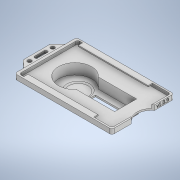
# Autodesk Inventor part: badge
Saved by Autodesk Inventor 2020 (Build 240168000, 168)
## iProperties
Created: 2019-12-22
Part Number: badge
Material: Generic
Document SubType Name: Modeling
Designer: user
Density: 1 g/cm^3
Appearance: Default
Author: user
## iProperties of the stored document _3DPrint.ipt
Created: 2019-12-23
Part Number: _3DPrint
Material: Generic
Document SubType Name: Modeling
Designer: user
Density: 1 g/cm^3
Appearance: Default
Author: user
Autodesk Inventor part; units mm, degrees
ref_plane "YZ Plane" through (0, 0, 0) normal (1, 0, 0) x (0, 1, 0)
ref_plane "XZ Plane" through (0, 0, 0) normal (0, 1, 0) x (-1, 0, 0)
ref_plane "XY Plane" through (0, 0, 0) normal (0, 0, 1) x (1, 0, 0)
sketch "Sketch1" plane through (0, 0, 0) normal (0, 1, 0) x (-1, 0, 0)
  line L0 (11.118, 24.1263) -> (-75.7851, 24.1263)
  line L1 (-75.7851, -33.7737) -> (11.118, -33.7737)
  line L2 (13.118, 15.5763) -> (20.4648, 8.8849)
  line L3 (21.118, 7.4063) -> (21.118, -16.3891)
  line L4 (20.5328, -17.8027) -> (13.118, -25.2237)
  line L5 (18.618, -9.3889) -> (18.618, 0.3517)
  circle A0 centre (-14.3851, -4.8237) radius 17
  line L6 (-63.1708, 4.9263) -> (-63.1708, -14.5737)
  line L7 (-61.1708, -16.5737) -> (-26.6708, -16.5737)
  line L8 (-26.6708, 6.9263) -> (-61.1708, 6.9263)
  arc A1 (-63.1708, -14.5737) -> (-61.1708, -16.5737) centre (-61.1708, -14.5737) ccw
  arc A2 (-61.1708, 6.9263) -> (-63.1708, 4.9263) centre (-61.1708, 4.9263) ccw
  line L9 (-29.1351, -0.5737) -> (-55.6708, -0.5737)
  line L10 (-55.6708, -0.5737) -> (-55.6708, -9.0737)
  line L11 (-55.6708, -9.0737) -> (-29.1351, -9.0737)
  line L12 (-29.1351, -9.0737) -> (-29.1351, -0.5737)
  line L13 (-77.7851, 6.1263) -> (-77.7851, 22.1263)
  line L14 (-77.7851, -15.7737) -> (-77.7851, -31.7737)
  line L15 (8.6149, 22.6263) -> (-74.2851, 22.6263)
  line L16 (-74.2851, -32.2737) -> (8.6149, -32.2737)
  line L17 (10.6149, -30.2737) -> (10.6149, 20.6263)
  line L18 (-76.2851, 20.6263) -> (-76.2851, 4.8009)
  line L19 (-76.2851, -30.2737) -> (-76.2851, -14.4482)
  line L20 (13.118, 22.1263) -> (13.118, 15.5763)
  line L21 (13.118, -25.2237) -> (13.118, -31.7737)
  arc A3 (-77.7851, -31.7737) -> (-75.7851, -33.7737) centre (-75.7851, -31.7737) ccw
  arc A4 (-76.2851, -30.2737) -> (-74.2851, -32.2737) centre (-74.2851, -30.2737) ccw
  arc A5 (-74.2851, 22.6263) -> (-76.2851, 20.6263) centre (-74.2851, 20.6263) ccw
  arc A6 (-75.7851, 24.1263) -> (-77.7851, 22.1263) centre (-75.7851, 22.1263) ccw
  arc A7 (13.118, 22.1263) -> (11.118, 24.1263) centre (11.118, 22.1263) ccw
  arc A8 (10.6149, 20.6263) -> (8.6149, 22.6263) centre (8.6149, 20.6263) ccw
  arc A9 (8.6149, -32.2737) -> (10.6149, -30.2737) centre (8.6149, -30.2737) ccw
  arc A10 (11.118, -33.7737) -> (13.118, -31.7737) centre (11.118, -31.7737) ccw
  arc A11 (20.5328, -17.8027) -> (21.118, -16.3891) centre (19.118, -16.3891) ccw
  arc A12 (21.118, 7.4063) -> (20.4648, 8.8849) centre (19.118, 7.4063) ccw
  arc A13 (-77.7851, -15.7737) -> (-77.7851, 6.1263) centre (-86.1254, -4.8237) ccw
  circle A14 centre (17.118, 6.2771) radius 1.8024
  circle A15 centre (17.118, -15.3502) radius 1.8024
  line L22 (13.118, 15.5763) -> (13.118, -25.2237)
  arc A16 (18.618, 0.3517) -> (15.618, 0.3153) centre (17.1248, -0.2229) ccw
  line L23 (15.618, 0.3153) -> (15.618, -9.4244)
  arc A17 (15.618, -9.4244) -> (18.618, -9.3889) centre (17.1115, -8.8502) ccw
  point P0 (0, 0)
  point P1 (13.118, 24.1263)
  point P2 (-77.7851, -33.7737)
  point P3 (-77.7851, 24.1263)
  point P4 (13.118, -33.7737)
  point P5 (21.118, -17.217)
  point P6 (-63.1708, -16.5737)
  dimension "d19" = 18
  dimension "d20" = 34
  dimension "d26" = 2
  dimension "d28" = 7.5
  dimension "d32" = 7.5
  dimension "d33" = 7.5
  dimension "d36" = 1.5
  dimension "d37" = 1.5
  dimension "d40" = 1.5
  dimension "d41" = 2
  dimension "d84" = 54.9
  dimension "d89" = 18
  dimension "d106" = 8
  dimension "d110" = 13.7646
  dimension "d116" = 1.5
  dimension "d122" = 3.6047
  dimension "d123" = 3.6047
  dimension "d155" = 25
  dimension "d163" = 15.7
  dimension "d164" = 15.7
  dimension "d165" = 27.45
  dimension "d166" = 27.45
  dimension "d167" = 8.5
  dimension "d171" = 26.5357
  dimension "d173" = 39.75
  dimension "d174" = 2.5032
  dimension "d177" = 86.9
  dimension "d182" = 4
  dimension "d183" = 4
  dimension "d187" = 3
  dimension "d188" = 1.6
  dimension "d189" = 1.6
  dimension "d190" = 2.5
  dimension "d191" = 2.5
  dimension "d192" = 8
  dimension "d193" = 6.5
  dimension "d194" = 6.5
  dimension "d195" = 6.55
  dimension "d196" = 6.55
  dimension "d202" = 15.7993
  dimension "d203" = 15.7993
  dimension "d204" = 23.7954
  dimension "d208" = 11.8273
  constraints: 48 end point, 34 point on circle, 24 tangent, 18 centre point, 13 point on line, 10 equal radius, 7 equal length, 5 vertical, 3 horizontal, 3 perpendicular
  measures "d19" distance of point (-77.785, 24.126) L13.start
  measures "d20" diameter of A0
  measures "d26" radius of A1
  measures "d28" distance between parallel lines of L7 L11
  measures "d32" distance between parallel lines of L9 L8
  measures "d33" distance between parallel lines of L6 L10
  measures "d36" distance between parallel lines of L0 L15
  measures "d37" distance between parallel lines of L1 L16
  measures "d40" distance between parallel lines of L14 L19
  measures "d41" radius of A3
  measures "d84" distance between parallel lines of L16 L15
  measures "d89" distance of L14.start point (-77.785, -33.774)
  measures "d106" distance between parallel lines of L20 L3
  measures "d110" radius of A13
  measures "d116" distance between parallel lines of L18 L13
  measures "d122" diameter of A15
  measures "d123" diameter of A14
  measures "d155" distance from line of L17 A0.centre
  measures "d163" distance between parallel lines of L16 L7
  measures "d164" distance between parallel lines of L15 L8
  measures "d165" distance from line of L16 A0.centre
  measures "d166" distance from line of L15 A0.centre
  measures "d167" distance between parallel lines of L9 L11
  measures "d171" distance between parallel lines of L10 L12
  measures "d173" distance between parallel lines of L17 L12
  measures "d174" distance between parallel lines of L17 L21
  measures "d177" distance between parallel lines of L19 L17
  measures "d182" distance from line of L22 A14.centre
  measures "d183" distance from line of L22 A15.centre
  measures "d187" distance between parallel lines of L23 L5
  measures "d188" radius of A16
  measures "d189" radius of A17
  measures "d190" distance between parallel lines of L3 L5
  measures "d191" distance between parallel lines of L22 L23
  measures "d192" distance between parallel lines of L22 L3
  measures "d193" distance of A14.centre A16.centre
  measures "d194" distance of A15.centre A17.centre
  measures "d195" distance of L20.start L2.start
  measures "d196" distance of L21.end L4.end
  measures "d202" vertical distance of L4.end L23.end
  measures "d203" vertical distance of L2.start A16.centre
  measures "d204" distance of L3.end L3.start
extrude "OutsideFrame_Ex" add sketch "Sketch1" along normal blind 4.5 contours A7 L20 L22 L21 A10 L1 A3 L14 A13 L19 A4 L16 A9 L17 A8 L15 A5 L18 L13 A6 L0
extrude "CardRidge" add sketch "Sketch1" along normal blind 1.5 contours L18 A5 L15 A8 L17 A9 L16 A4 L19 A13
extrude "TokenBuffer" add sketch "Sketch1" against normal blind 10 contours A0 L11 L12 L9 | A0 L9 L10 L11 L7 A1 L6 A2 L8 picked at (-18.5518, -4.8237)
sketch "Sketch4" plane through (0, 0, 0) normal (0, 1, 0) x (1, 0, 0)
  arc A0 (26.6708, 16.5737) -> (26.6708, -6.9263) centre (14.3851, 4.8237) ccw projected
  circle A1 centre (14.3851, 4.8237) radius 15.5
  line L0 (26.0122, -5.4263) -> (61.6708, -5.4263)
  line L1 (61.6708, -5.4263) -> (61.6708, 15.0737)
  line L2 (61.6708, 15.0737) -> (26.0122, 15.0737)
  line L3 (26.0122, 15.0737) -> (26.0122, -5.4263)
  line L4 (61.1708, -6.9263) -> (26.6708, -6.9263) projected
  line L5 (26.6708, 16.5737) -> (61.1708, 16.5737) projected
  line L6 (63.1708, 14.5737) -> (63.1708, -4.9263) projected
  point P0 (0, 0)
  point P1 (26.0122, 15.0737)
  point P2 (26.0122, 15.0737)
  dimension "d56" = 1.5
  dimension "d57" = 1.5
  dimension "d58" = 1.5
  dimension "d59" = 1.5
  constraints: 8 end point, 2 parallel, 1 coincident, 1 horizontal, 1 perpendicular, 3 other
  measures "d57" distance between parallel lines of L4 L0
  measures "d58" distance between parallel lines of L5 L2
  measures "d59" distance between parallel lines of L6 L1
extrude "TokenCut" cut sketch "Sketch4" against normal blind 8.5
sketch "Sketch5" plane through (74.2851, 4.5, 22.6263) normal (0, 0, -1) x (-1, 0, 0)
  line L0 (-2, 0) -> (0, 0) projected
  line L1 (80.4, 0) -> (80.4, -1)
  line L2 (0, 0) -> (82.9, 0) projected
  line L3 (15, 0) -> (80.4, 0)
  line L4 (80.4, 0) -> (80.4, -1)
  line L5 (80.4, -1) -> (15, -1)
  line L6 (15, -1) -> (15, 0)
  line L7 (0, -4.5) -> (0, 0) projected
  line L8 (82.9, -4.5) -> (82.9, 0) projected
  line L9 (0, -3) -> (82.9, -3) projected
  point P0 (74.2851, -4.5)
  dimension "d65" = 15
  dimension "d66" = 2.5
  dimension "d67" = 1
  constraints: 10 end point, 2 parallel, 1 horizontal, 1 perpendicular, 1 point on line
  measures "d65" distance between parallel lines of L7 L6
  measures "d66" distance between parallel lines of L8 L1
  measures "d67" distance between parallel lines of L5 L2
extrude "LeftSlider" add sketch "Sketch5" along normal blind 4 contours L1 L5 L6 L2
sketch "Sketch6" plane through (-8.6149, 4.5, -32.2737) normal (0, 0, 1) x (1, 0, 0)
  line L0 (84.4, 0) -> (-2.5032, 0) projected
  line L1 (2.5, 0) -> (67.9, 0)
  line L2 (67.9, 0) -> (67.9, -1)
  line L3 (67.9, -1) -> (2.5, -1)
  line L4 (2.5, -1) -> (2.5, 0)
  line L5 (0, -3) -> (0, 0) projected
  line L6 (82.9, -3) -> (82.9, 0) projected
  point P0 (8.6149, -4.5)
  point P1 (0, -7.4)
  point P2 (83.7968, -7.4)
  dimension "d71" = 2.5
  dimension "d72" = 15
  dimension "d73" = 1
  constraints: 8 end point, 2 parallel, 1 horizontal, 1 perpendicular, 1 point on line, 1 other
  measures "d71" distance between parallel lines of L5 L4
  measures "d73" distance between parallel lines of L3 L0
extrude "RightSlider" add sketch "Sketch6" along normal blind 4
sketch "Sketch12" plane through (0, 0, 0) normal (0, 1, 0) x (1, 0, 0)
  arc A0 (26.0122, 15.0737) -> (26.0122, -5.4263) centre (14.3851, 4.8237) ccw projected
  circle A1 centre (14.3851, 4.8237) radius 15.5
  line L0 (61.1708, -6.9263) -> (26.6708, -6.9263) projected
  line L1 (26.6708, -6.9263) -> (61.1708, -6.9263)
  line L2 (63.1708, 14.5737) -> (63.1708, -4.9263) projected
  arc A2 (61.1708, -6.9263) -> (63.1708, -4.9263) centre (61.1708, -4.9263) ccw
  line L3 (61.6708, -5.4263) -> (26.0122, -5.4263) projected
  line L4 (26.0122, -5.4263) -> (61.6708, -5.4263)
  line L5 (61.6708, 15.0737) -> (61.6708, -5.4263) projected
  line L6 (61.6708, -5.4263) -> (61.6708, 15.0737)
  line L7 (26.0122, 15.0737) -> (61.6708, 15.0737) projected
  line L8 (61.6708, 15.0737) -> (26.0122, 15.0737)
  line L9 (63.1708, -4.9263) -> (63.6141, 19.5737)
  line L10 (63.1708, 14.5737) -> (63.1708, -4.9263) projected
  line L11 (63.1708, -4.9263) -> (63.1708, 14.5737)
  line L12 (26.6708, 16.5737) -> (61.1708, 16.5737) projected
  arc A3 (63.1708, 14.5737) -> (61.1708, 16.5737) centre (61.1708, 14.5737) ccw
  line L13 (61.1708, 16.5737) -> (26.6708, 16.5737)
  circle A4 centre (14.3851, 4.8237) radius 17
  point P0 (0, 0)
  point P1 (26.6708, 16.5737)
  dimension "d152" = 34
  constraints: 14 end point, 4 centre point, 4 point on circle, 2 coincident, 2 horizontal, 2 perpendicular, 1 collinear, 1 tangent
  measures "d152" diameter of A4
sketch "Sketch15" plane through (77.7851, 0, -15.7737) normal (1, 0, 0) x (0, 0, -1)
  line L0 (1.9095, 3.8757) -> (15.579, 3.8757) construction
  line L1 (15.579, 3.8757) -> (15.579, 0.6243) construction
  line L2 (15.579, 0.6243) -> (1.9095, 0.6243) construction
  line L3 (1.9095, 0.6243) -> (1.9095, 3.8757) construction
  line L4 (0, 4.5) -> (16, 4.5) projected
  line L5 (0, 0) -> (16, 0) projected
  line L6 (3.9843, 3.0532) -> (3.1223, 0.766)
  line L7 (3.1223, 0.766) -> (2.7765, 0.766)
  line L8 (2.7765, 0.766) -> (1.9218, 3.0532)
  line L9 (1.9218, 3.0532) -> (2.3393, 3.0532)
  line L10 (2.3393, 3.0532) -> (2.9642, 1.2921)
  line L11 (2.9642, 1.2921) -> (3.5842, 3.0532)
  line L12 (3.5842, 3.0532) -> (3.9843, 3.0532)
  line L13 (5.9455, 0.766) -> (4.4586, 0.766)
  line L14 (4.4586, 0.766) -> (4.4586, 1.0772)
  line L15 (4.4586, 1.0772) -> (5.0118, 1.0772)
  line L16 (5.0118, 1.0772) -> (5.0118, 3.1199)
  line L17 (5.0118, 3.1199) -> (4.4586, 3.1199)
  line L18 (4.4586, 3.1199) -> (4.4586, 3.399)
  spline S0 degree 2 poles (4.4586, 3.399) (4.7722, 3.399) (5.0686, 3.5769) (5.0884, 3.8239) knots 0 0 0 1 2 2 2
  line L19 (5.0884, 3.8239) -> (5.4046, 3.8239)
  line L20 (5.4046, 3.8239) -> (5.4046, 1.0772)
  line L21 (5.4046, 1.0772) -> (5.9455, 1.0772)
  line L22 (5.9455, 1.0772) -> (5.9455, 0.766)
  line L23 (7.1608, 0.766) -> (6.6717, 0.766)
  line L24 (6.6717, 0.766) -> (6.6717, 1.3489)
  line L25 (6.6717, 1.3489) -> (7.1608, 1.3489)
  line L26 (7.1608, 1.3489) -> (7.1608, 0.766)
  spline S1 degree 2 poles (9.6728, 2.29) (9.6728, 1.4699) (9.196, 0.7018) (8.6996, 0.7018) knots 0 0 0 1 2 2 2
  spline S2 degree 2 poles (8.6996, 0.7018) (8.1957, 0.7018) (7.7239, 1.4848) (7.7239, 2.2875) knots 0 0 0 1 2 2 2
  spline S3 degree 2 poles (7.7239, 2.2875) (7.7239, 3.1125) (8.2006, 3.8757) (8.6996, 3.8757) knots 0 0 0 1 2 2 2
  spline S4 degree 2 poles (8.6996, 3.8757) (9.201, 3.8757) (9.6728, 3.0853) (9.6728, 2.29) knots 0 0 0 1 2 2 2
  spline S5 degree 2 poles (9.1491, 1.3612) (9.2084, 1.5119) (9.2578, 1.9763) (9.2578, 2.29) knots 0 0 0 1 2 2 2
  spline S6 degree 2 poles (9.2578, 2.29) (9.2578, 2.6037) (9.2084, 3.0656) (9.1466, 3.2212) knots 0 0 0 1 2 2 2
  spline S7 degree 2 poles (9.1466, 3.2212) (9.0849, 3.3768) (8.87, 3.5373) (8.6996, 3.5373) knots 0 0 0 1 2 2 2
  spline S8 degree 2 poles (8.6996, 3.5373) (8.5291, 3.5373) (8.3093, 3.3768) (8.2451, 3.2162) knots 0 0 0 1 2 2 2
  spline S9 degree 2 poles (8.2451, 3.2162) (8.1833, 3.0606) (8.1389, 2.5864) (8.1389, 2.2875) knots 0 0 0 1 2 2 2
  spline S10 degree 2 poles (8.1389, 2.2875) (8.1389, 1.9664) (8.1784, 1.5366) (8.2426, 1.3687) knots 0 0 0 1 2 2 2
  spline S11 degree 2 poles (8.2426, 1.3687) (8.3019, 1.2106) (8.5217, 1.0401) (8.6996, 1.0401) knots 0 0 0 1 2 2 2
  spline S12 degree 2 poles (8.6996, 1.0401) (8.8675, 1.0401) (9.0874, 1.2007) (9.1491, 1.3612) knots 0 0 0 1 2 2 2
  line L27 (10.7176, 0.766) -> (10.2285, 0.766)
  line L28 (10.2285, 0.766) -> (10.2285, 1.3489)
  line L29 (10.2285, 1.3489) -> (10.7176, 1.3489)
  line L30 (10.7176, 1.3489) -> (10.7176, 0.766)
  spline S13 degree 2 poles (11.2486, 2.8235) (11.2486, 3.0582) (11.4018, 3.4484) (11.5351, 3.5892) knots 0 0 0 1 2 2 2
  spline S14 degree 2 poles (11.5351, 3.5892) (11.6611, 3.7251) (12.0292, 3.8757) (12.2169, 3.8757) knots 0 0 0 1 2 2 2
  spline S15 degree 2 poles (12.2169, 3.8757) (12.4268, 3.8757) (12.7677, 3.7349) (12.8937, 3.6016) knots 0 0 0 1 2 2 2
  spline S16 degree 2 poles (12.8937, 3.6016) (13.0517, 3.4336) (13.2246, 2.8902) (13.2246, 2.4728) knots 0 0 0 1 2 2 2
  spline S17 degree 2 poles (13.2246, 2.4728) (13.2246, 2.0948) (13.0542, 1.4181) (12.8887, 1.1933) knots 0 0 0 1 2 2 2
  spline S18 degree 2 poles (12.8887, 1.1933) (12.7133, 0.9562) (12.2193, 0.7067) (11.8587, 0.7067) knots 0 0 0 1 2 2 2
  spline S19 degree 2 poles (11.8587, 0.7067) (11.7772, 0.7067) (11.592, 0.724) (11.5129, 0.7487) knots 0 0 0 1 2 2 2
  line L31 (11.5129, 0.7487) -> (11.5129, 1.1414)
  line L32 (11.5129, 1.1414) -> (11.5327, 1.1414)
  spline S20 degree 2 poles (11.5327, 1.1414) (11.5846, 1.1118) (11.8019, 1.0599) (11.9131, 1.0599) knots 0 0 0 1 2 2 2
  spline S21 degree 2 poles (11.9131, 1.0599) (12.3132, 1.0599) (12.7702, 1.5885) (12.8023, 2.0776) knots 0 0 0 1 2 2 2
  spline S22 degree 2 poles (12.8023, 2.0776) (12.6392, 1.9664) (12.3428, 1.8651) (12.1675, 1.8651) knots 0 0 0 1 2 2 2
  spline S23 degree 2 poles (12.1675, 1.8651) (11.9995, 1.8651) (11.7204, 1.9392) (11.5796, 2.0454) knots 0 0 0 1 2 2 2
  spline S24 degree 2 poles (11.5796, 2.0454) (11.4166, 2.1714) (11.2486, 2.5543) (11.2486, 2.8235) knots 0 0 0 1 2 2 2
  spline S25 degree 2 poles (12.8121, 2.5641) (12.8121, 2.8729) (12.6985, 3.2632) (12.5973, 3.3694) knots 0 0 0 1 2 2 2
  spline S26 degree 2 poles (12.5973, 3.3694) (12.5083, 3.4682) (12.3231, 3.5423) (12.2144, 3.5423) knots 0 0 0 1 2 2 2
  spline S27 degree 2 poles (12.2144, 3.5423) (11.9625, 3.5423) (11.6636, 3.1817) (11.6636, 2.8408) knots 0 0 0 1 2 2 2
  spline S28 degree 2 poles (11.6636, 2.8408) (11.6636, 2.6481) (11.7624, 2.3987) (11.8711, 2.3097) knots 0 0 0 1 2 2 2
  spline S29 degree 2 poles (11.8711, 2.3097) (11.9501, 2.2455) (12.1452, 2.2035) (12.2589, 2.2035) knots 0 0 0 1 2 2 2
  spline S30 degree 2 poles (12.2589, 2.2035) (12.3898, 2.2035) (12.6911, 2.2949) (12.8047, 2.3715) knots 0 0 0 1 2 2 2
  spline S31 degree 2 poles (12.8047, 2.3715) (12.8072, 2.4011) (12.8121, 2.5024) (12.8121, 2.5641) knots 0 0 0 1 2 2 2
  point P0 (-15.7737, 0)
  dimension "d178" = 0.6243
  dimension "d179" = 0.6243
  constraints: 2 other
  measures "d178" distance between parallel lines of L4 L0
  measures "d179" distance between parallel lines of L5 L2
emboss "VersionNumber" sketch "Sketch15" operation cut depth 1 direction (-1, 0, 0)
extrude "Extrusion15" add sketch "Sketch1" along normal blind 3.5 contours L2 A12 L3 A11 L4 L22
extrude "Extrusion16" cut sketch "Sketch1" along normal blind 1 contours L2 A12 L3 A11 L4 L22 | A17 L23 A16 L5
extrude "Extrusion17" add sketch "Sketch12" along normal blind 1.5 contours A0 L3 A4 L7 | A4 L12 A3 L2 A2 L0 L3 L5 L7
sketch "Sketch22" plane through (0, -8.5, 0) normal (0, 1, 0) x (1, 0, 0)
  circle A0 centre (17.3851, 4.8237) radius 9
  arc A1 (26.0122, 15.0737) -> (26.0122, -5.4263) centre (14.3851, 4.8237) ccw projected
  point P0 (0, 0)
  dimension "d215" = 0
  dimension "d216" = 18
  dimension "d217" = 3
  constraints: 1 centre point
  measures "d215" vertical distance of A1.centre A0.centre
  measures "d216" diameter of A0
  measures "d217" distance of A0.centre A1.centre
extrude "Extrusion19" cut sketch "Sketch22" against normal blind 0.75
fillet "Fillet6" radius 2 1 edges at (8.3851, -8.5, -4.8237)
equation "\"d89\" = d19"
body "Solid3"
